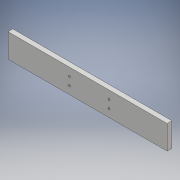
# Autodesk Inventor part: Placa do Circuito
Saved by Autodesk Inventor 2018 (Build 220112000, 112)
## iProperties
Created: 2018-02-27
Part Number: Placa do Circuito
Material: Generic
Document SubType Name: Modeling
Designer: matheus
Density: 1 g/cm^3
Appearance: Default
Author: matheus
Autodesk Inventor part; units mm, degrees
ref_plane "YZ Plane" through (0, 0, 0) normal (1, 0, 0) x (0, 1, 0)
ref_plane "XZ Plane" through (0, 0, 0) normal (0, 1, 0) x (-1, 0, 0)
ref_plane "XY Plane" through (0, 0, 0) normal (0, 0, 1) x (1, 0, 0)
sketch "Sketch1" plane through (0, 0, 0) normal (0, 1, 0) x (-1, 0, 0)
  line L0 (-50, 7.5) -> (50, 7.5)
  line L1 (50, 7.5) -> (50, -7.5)
  line L2 (50, -7.5) -> (-50, -7.5)
  line L3 (-50, -7.5) -> (-50, 7.5)
  point P0 (0, 0)
  dimension "d2" = 100
  dimension "d3" = 15
  constraints: 8 end point, 2 parallel, 1 horizontal, 1 perpendicular
  measures "d2" distance of L1.end L2.end
  measures "d3" distance of L0.end L1.end
extrude "Extrusion1" add sketch "Sketch1" along normal blind 3
sketch "Sketch2" plane through (0, 0, 0) normal (0, -1, 0) x (1, 0, 0)
  line L0 (13.0431, 2.8913) -> (14.0431, 2.8913)
  line L1 (14.0431, 2.8913) -> (14.0431, 1.8913)
  line L2 (14.0431, 1.8913) -> (13.0431, 1.8913)
  line L3 (13.0431, 1.8913) -> (13.0431, 2.8913)
  line L4 (13.0431, -2.1087) -> (14.0431, -2.1087)
  line L5 (14.0431, -2.1087) -> (14.0431, -3.1087)
  line L6 (14.0431, -3.1087) -> (13.0431, -3.1087)
  line L7 (13.0431, -3.1087) -> (13.0431, -2.1087)
  line L8 (-10.9569, 1.8913) -> (-11.9569, 1.8913)
  line L9 (-11.9569, 1.8913) -> (-11.9569, 2.8913)
  line L10 (-11.9569, 2.8913) -> (-10.9569, 2.8913)
  line L11 (-10.9569, 2.8913) -> (-10.9569, 1.8913)
  line L12 (-10.9569, -2.1087) -> (-11.9569, -2.1087)
  line L13 (-11.9569, -2.1087) -> (-11.9569, -3.1087)
  line L14 (-11.9569, -3.1087) -> (-10.9569, -3.1087)
  line L15 (-10.9569, -3.1087) -> (-10.9569, -2.1087)
  point P0 (0, 0)
  dimension "d7" = 1
  dimension "d8" = 4
  dimension "d9" = 1
  dimension "d10" = 1
  dimension "d11" = 24
  dimension "d12" = 1
  dimension "d13" = 1
  dimension "d14" = 4
  dimension "d15" = 1
  dimension "d16" = 1
  constraints: 32 end point, 8 parallel, 4 horizontal, 4 perpendicular
  measures "d7" distance of L0.end L1.end
  measures "d8" distance of L2.end L4.start
  measures "d9" distance of L5.end L6.end
  measures "d10" distance of L4.end L5.end
  measures "d11" distance of L2.end L8.start
  measures "d12" distance of L9.end L10.end
  measures "d13" distance of L8.end L9.end
  measures "d14" distance of L8.start L12.start
  measures "d15" distance of L14.end L13.end
  measures "d16" distance of L13.end L12.end
extrude "Extrusion2" cut sketch "Sketch2" along normal mid plane 10
body "Solid1"
